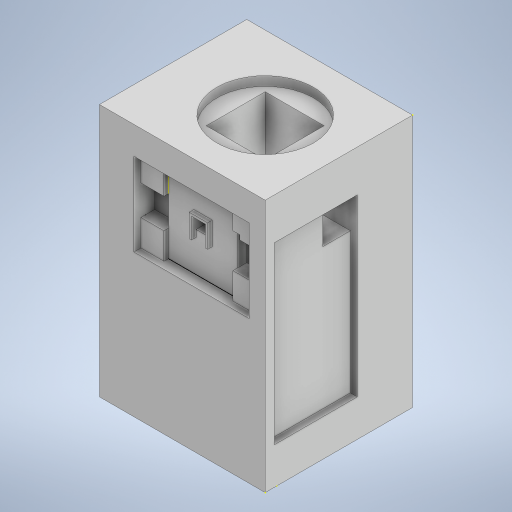
# Autodesk Inventor part: Cuvette Holder v2
Saved by Autodesk Inventor 2024 (Build 280153000, 153)
## iProperties
Created: 2023-06-29
Part Number: Cuvette Holder v2
Material: Generic
Document SubType Name: Modeling
Designer: Russe
Density: 1 g/cm^3
Appearance: Default
Author: Russe
Autodesk Inventor part; units mm, degrees
ref_plane "YZ Plane" through (0, 0, 0) normal (1, 0, 0) x (0, 1, 0)
ref_plane "XZ Plane" through (0, 0, 0) normal (0, 1, 0) x (-1, 0, 0)
ref_plane "XY Plane" through (0, 0, 0) normal (0, 0, 1) x (1, 0, 0)
sketch "Sketch1" plane through (0, 0, 0) normal (0, 1, 0) x (-1, 0, 0)
  line L0 (32, 32) -> (0, 32)
  line L1 (0, 32) -> (0, 0)
  line L2 (0, 0) -> (32, 0)
  line L3 (32, 0) -> (32, 32)
  constraints: 8 end point, 2 parallel, 1 horizontal, 1 perpendicular
extrude "Extrusion1" add sketch "Sketch1" along normal blind 55
sketch "Sketch2" plane through (0, 55, 0) normal (0, 1, 0) x (1, 0, 0)
  line L0 (-9.6, -9.6) -> (-22.4, -9.6)
  line L1 (-22.4, -9.6) -> (-22.4, -22.4)
  line L2 (-22.4, -22.4) -> (-9.6, -22.4)
  line L3 (-9.6, -22.4) -> (-9.6, -9.6)
  point P0 (0, 0)
  constraints: 8 end point, 2 parallel, 1 horizontal, 1 perpendicular
extrude "Extrusion2" cut sketch "Sketch2" against normal blind 30
sketch "Sketch3" plane through (-32, 0, 32) normal (0, 0, 1) x (1, 0, 0)
  line L0 (3.5, 49) -> (28.5, 49)
  line L1 (28.5, 49) -> (28.5, 31)
  line L2 (28.5, 31) -> (3.5, 31)
  line L3 (3.5, 31) -> (3.5, 49)
  line L4 (3.5, 49) -> (3.5, 43.25)
  line L5 (3.5, 36.75) -> (3.5, 43.25)
  line L6 (28.5, 49) -> (28.5, 43.25)
  line L7 (28.5, 36.75) -> (28.5, 43.25)
  line L8 (3.5, 43.25) -> (3.5, 36.75)
  line L9 (28.5, 43.25) -> (28.5, 36.75)
  point P0 (32, 0)
  constraints: 20 end point, 2 collinear, 2 parallel, 1 horizontal, 1 perpendicular
extrude "Extrusion3" cut sketch "Sketch3" against normal blind 2.5
sketch "Sketch4" plane through (-32, 0, 29.5) normal (0, 0, 1) x (1, 0, 0)
  line L0 (3.5, 49) -> (28.5, 49) projected
  line L1 (3.5, 49) -> (3.5, 43.25)
  line L2 (28.5, 31) -> (3.5, 31) projected
  line L3 (3.5, 36.75) -> (3.5, 31)
  line L4 (3.5, 31) -> (28.5, 31)
  line L5 (28.5, 31) -> (28.5, 36.75)
  line L6 (28.5, 49) -> (28.5, 31) projected
  line L7 (28.5, 43.25) -> (28.5, 49)
  line L8 (28.5, 49) -> (3.5, 49)
  point P0 (32, 0)
  constraints: 12 end point, 4 perpendicular, 2 collinear
sketch "Sketch5" plane through (-32, 0, 29.5) normal (0, 0, 1) x (1, 0, 0)
  line L0 (3.5, 43.25) -> (8.5, 43.25)
  line L1 (8.5, 43.25) -> (8.5, 36.75)
  line L2 (8.5, 36.75) -> (3.5, 36.75)
  line L3 (3.5, 36.75) -> (3.5, 43.25)
  point P0 (32, 0)
  constraints: 8 end point, 2 parallel, 1 horizontal, 1 perpendicular
sketch "Sketch6" plane through (-32, 0, 29.5) normal (0, 0, 1) x (1, 0, 0)
  line L0 (28.5, 43.25) -> (23.5, 43.25)
  line L1 (23.5, 43.25) -> (23.5, 36.75)
  line L2 (23.5, 36.75) -> (28.5, 36.75)
  line L3 (28.5, 36.75) -> (28.5, 43.25)
  point P0 (32, 0)
  constraints: 8 end point, 2 parallel, 1 horizontal, 1 perpendicular
extrude "Extrusion4" cut sketch "Sketch5" against normal blind 2
extrude "Extrusion5" cut sketch "Sketch6" against normal blind 2
sketch "Sketch7" plane through (-32, 0, 29.5) normal (0, 0, 1) x (1, 0, 0)
  line L0 (3.5, 43.25) -> (8.5, 43.25) projected
  line L1 (3.5, 43.25) -> (3.5, 49) projected
  line L2 (8.5, 43.25) -> (3.5, 43.25)
  line L3 (3.5, 43.25) -> (3.5, 49)
  line L4 (3.5, 49) -> (8.5, 49)
  line L5 (8.5, 49) -> (8.5, 43.25)
  point P0 (32, 0)
  constraints: 8 end point, 2 parallel, 1 horizontal, 1 perpendicular
sketch "Sketch8" plane through (-32, 0, 29.5) normal (0, 0, 1) x (1, 0, 0)
  line L0 (8.5, 36.75) -> (3.5, 36.75) projected
  line L1 (28.5, 31) -> (3.5, 31) projected
  line L2 (8.5, 36.75) -> (3.5, 36.75)
  line L3 (3.5, 36.75) -> (3.5, 31)
  line L4 (3.5, 31) -> (8.5, 31)
  line L5 (8.5, 31) -> (8.5, 36.75)
  point P0 (32, 0)
  constraints: 8 end point, 2 parallel, 1 horizontal, 1 perpendicular
sketch "Sketch9" plane through (-32, 0, 29.5) normal (0, 0, 1) x (1, 0, 0)
  line L0 (28.5, 36.75) -> (23.5, 36.75) projected
  line L1 (28.5, 31) -> (3.5, 31) projected
  line L2 (23.5, 36.75) -> (28.5, 36.75)
  line L3 (28.5, 36.75) -> (28.5, 31)
  line L4 (28.5, 31) -> (23.5, 31)
  line L5 (23.5, 31) -> (23.5, 36.75)
  point P0 (32, 0)
  constraints: 8 end point, 2 parallel, 1 horizontal, 1 perpendicular
sketch "Sketch10" plane through (-32, 0, 29.5) normal (0, 0, 1) x (1, 0, 0)
  line L0 (23.5, 43.25) -> (28.5, 43.25) projected
  line L1 (28.5, 49) -> (28.5, 43.25) projected
  line L2 (23.5, 43.25) -> (28.5, 43.25)
  line L3 (28.5, 43.25) -> (28.5, 49)
  line L4 (28.5, 49) -> (23.5, 49)
  line L5 (23.5, 49) -> (23.5, 43.25)
  point P0 (32, 0)
  constraints: 8 end point, 2 parallel, 1 horizontal, 1 perpendicular
extrude "Extrusion6" add sketch "Sketch7" along normal blind 1
extrude "Extrusion7" add sketch "Sketch8" along normal blind 1
extrude "Extrusion8" add sketch "Sketch9" along normal blind 1
extrude "Extrusion9" add sketch "Sketch10" along normal blind 1
sketch "Sketch11" plane through (-32, 0, 30.5) normal (0, 0, 1) x (1, 0, 0)
  line L0 (23.5, 43.25) -> (28.5, 43.25) projected
  line L1 (23.5, 43.25) -> (25, 43.25)
  line L2 (25, 43.25) -> (25, 44.25)
  line L3 (25, 44.25) -> (23.5, 44.25)
  line L4 (23.5, 44.25) -> (23.5, 43.25)
  point P0 (32, 0)
  constraints: 8 end point, 2 parallel, 1 horizontal, 1 perpendicular
extrude "Extrusion10" cut sketch "Sketch11" against normal blind 1
sketch "Sketch12" plane through (-32, 0, 29.5) normal (0, 0, 1) x (1, 0, 0)
  line L0 (8.5, 49) -> (8.5, 43.25) projected
  line L1 (23.5, 31) -> (8.5, 31) projected
  line L2 (23.5, 49) -> (23.5, 44.25) projected
  point P0 (32, 0)
sketch "Sketch13" plane through (-32, 0, 29.5) normal (0, 0, 1) x (1, 0, 0)
  point P0 (32, 0)
sketch "Sketch14" plane through (-32, 0, 29.5) normal (0, 0, 1) x (1, 0, 0)
  line L0 (23.5, 44.25) -> (23.5, 49) projected
  line L1 (23.5, 49) -> (17.5, 49)
  line L2 (14.5, 43) -> (17.5, 43)
  line L3 (17.5, 38) -> (18, 38)
  line L4 (18, 38) -> (18, 43)
  line L5 (18, 43) -> (14, 43)
  line L6 (14, 43) -> (14, 38)
  line L7 (14, 38) -> (14.5, 38)
  line L8 (14.5, 38) -> (14.5, 42)
  line L9 (3.5, 43.25) -> (8.5, 43.25) projected
  line L10 (14.5, 42) -> (14.5, 42.5)
  line L11 (14.5, 42.5) -> (17.5, 42.5)
  line L12 (17.5, 42.5) -> (17.5, 38)
  point P0 (32, 0)
  constraints: 22 end point, 3 perpendicular, 2 collinear, 1 horizontal
extrude "Extrusion11" add sketch "Sketch14" along normal blind 1
sketch "Sketch15" plane through (-32, 0, 29.5) normal (0, 0, 1) x (1, 0, 0)
  line L0 (14.5, 42.5) -> (14.5, 38) projected
  line L1 (14.5, 42.5) -> (17.5, 42.5)
  line L2 (17.5, 42.5) -> (17.5, 39.5)
  line L3 (17.5, 39.5) -> (14.5, 39.5)
  line L4 (14.5, 39.5) -> (14.5, 42.5)
  point P0 (32, 0)
  constraints: 8 end point, 2 parallel, 1 horizontal, 1 perpendicular
extrude "Extrusion12" cut sketch "Sketch15" against normal blind 7.1
sketch "Sketch16" plane through (-32, 0, 32) normal (0, 0, 1) x (1, 0, 0)
  point P0 (32, 0)
sketch "Sketch17" plane through (0, 0, 32) normal (1, 0, 0) x (0, 0, -1)
  line L0 (2, 46) -> (20, 46)
  line L1 (20, 46) -> (20, 8)
  line L2 (20, 8) -> (2, 8)
  line L3 (2, 8) -> (2, 46)
  point P0 (32, 0)
  constraints: 8 end point, 2 parallel, 1 horizontal, 1 perpendicular
extrude "Extrusion13" cut sketch "Sketch17" against normal blind 1.5
sketch "Sketch18" plane through (-1.5, 0, 32) normal (1, 0, 0) x (0, 0, -1)
  line L0 (20, 38.5) -> (14, 38.5)
  line L1 (14, 38.5) -> (14, 46)
  line L2 (14, 46) -> (20, 46)
  line L3 (20, 46) -> (20, 38.5)
  point P0 (32, 0)
  constraints: 8 end point, 2 parallel, 1 horizontal, 1 perpendicular
extrude "Extrusion14" cut sketch "Sketch18" against normal blind 8.1
sketch "Sketch19" plane through (0, 55, 0) normal (0, 1, 0) x (1, 0, 0)
  circle A0 centre (-16, -16) radius 10.5
  point P0 (0, 0)
  constraints: 1 centre point
sketch "Sketch20" plane through (0, 55, 0) normal (0, 1, 0) x (1, 0, 0)
  point P0 (0, 0)
extrude "Extrusion15" cut sketch "Sketch19" against normal blind 2
sketch "Sketch21" plane through (-32, 0, 0) normal (-1, 0, 0) x (0, 0, 1)
  line L0 (32, 0) -> (32, 55) projected
  line L1 (0, 0) -> (32, 0)
  line L2 (32, 0) -> (32, 55)
  line L3 (32, 55) -> (0, 55)
  line L4 (0, 55) -> (0, 0)
  constraints: 8 end point, 2 parallel, 1 horizontal, 1 perpendicular
extrude "Extrusion16" add sketch "Sketch21" along normal blind 4
sketch "Sketch22" plane through (-36, 0, 0) normal (-1, 0, 0) x (0, 0, 1)
  line L0 (2, 3) -> (4, 3)
  line L1 (4, 3) -> (4, 52)
  line L2 (4, 52) -> (2, 52)
  line L3 (2, 52) -> (2, 3)
  line L4 (23, 3) -> (25, 3)
  line L5 (25, 3) -> (25, 52)
  line L6 (25, 52) -> (23, 52)
  line L7 (23, 52) -> (23, 3)
  point P0 (0, 0)
  constraints: 16 end point, 4 parallel, 2 horizontal, 2 perpendicular
extrude "Extrusion17" cut sketch "Sketch22" against normal blind 11
body "Solid1"
